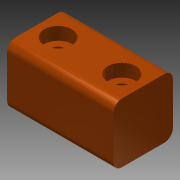
# Autodesk Inventor part: string tensioner
Saved by Autodesk Inventor 2013 (Build 170138000, 138)
## iProperties
Created: 2013-08-04
Part Number: string tensioner
Material: Generic
Document SubType Name: Modeling
Designer: employee
Density: 1 g/cm^3
Mass: 4.44901 g
Surface Area: 20.0588 cm^2
Volume: 4.44901 cm^3
Author: employee
Autodesk Inventor part; units mm, degrees
ref_plane "YZ Plane" through (0, 0, 0) normal (1, 0, 0) x (0, 1, 0)
ref_plane "XZ Plane" through (0, 0, 0) normal (0, 1, 0) x (-1, 0, 0)
ref_plane "XY Plane" through (0, 0, 0) normal (0, 0, 1) x (1, 0, 0)
sketch "Sketch1" plane through (0, 0, 0) normal (0, 0, 1) x (1, 0, 0)
  line L0 (-12.5, 7) -> (12.5, 7)
  line L1 (12.5, 7) -> (12.5, -7)
  line L2 (12.5, -7) -> (-12.5, -7)
  line L3 (-12.5, -7) -> (-12.5, 7)
  point P0 (0, 0)
  point P1 (12.5, 0)
  point P2 (0, 7)
  dimension "d0" = 25
  dimension "d2" = 14
  constraints: 8 end point, 2 midpoint, 2 parallel, 1 horizontal, 1 horizontal alignment, 1 perpendicular, 1 vertical alignment
  measures "d0" distance of L1.end L2.end
  measures "d2" distance of L0.end L1.end
extrude "Extrusion1" add sketch "Sketch1" along normal blind 14
sketch "Sketch2" plane through (0, 0, 14) normal (0, 0, 1) x (1, 0, 0)
  line L0 (-7.5, 0) -> (7.5, 0)
  point P0 (0, 0)
  point P1 (0, 0)
  dimension "d5" = 15
  constraints: 2 end point, 1 coincident, 1 horizontal, 1 midpoint
  measures "d5" distance of L0.start L0.end
hole "Hole1" at (-7.5, 0, 14) at (7.5, 0, 14) direction (0, 0, -1) diameter 3.1 end through all counterbore diameter 6.5 counterbore depth 3 clearance for "Socket Head Cap Screw" size "M3" standard "Ansi Metric M Profile"
fillet "Fillet1" radius 2 2 edges at (0, 7, 0) (0, -7, 0)
fillet "Fillet2" radius 2 2 edges at (0, 7, 14) (0, -7, 14)
body "Solid1"
